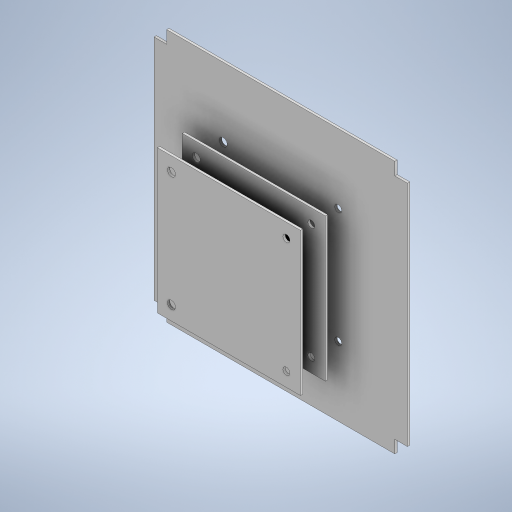
# Autodesk Inventor part: PCB_COM_BAT
Saved by Autodesk Inventor 2024 (Build 280153000, 153)
## iProperties
Created: 2023-06-28
Part Number: PCB_COM_BAT
Material: Genérico
Document SubType Name: Modeling
Designer: Personal
Density: 3.19616 g/cm^3
Appearance: Valor por defecto
Mass: 277 g
Surface Area: 1079.17 cm^2
Volume: 86.6665 cm^3
Author: Personal
Autodesk Inventor part; units mm, degrees
ref_plane "YZ Plane" through (0, 0, 0) normal (1, 0, 0) x (0, 1, 0)
sketch "Boceto1" plane through (0, 0, 0) normal (0, 0, 1) x (1, 0, 0)
  line L0 (-121.9033, -49.2033) -> (40.2033, -49.2033) projected
  line L1 (40.2033, -49.2033) -> (40.2033, -40.2033) projected
  line L2 (40.2033, -40.2033) -> (49.2033, -40.2033) projected
  line L3 (49.2033, -40.2033) -> (49.2033, 121.9033) projected
  line L4 (49.2033, 121.9033) -> (40.2033, 121.9033) projected
  line L5 (40.2033, 121.9033) -> (40.2033, 130.9033) projected
  line L6 (40.2033, 130.9033) -> (-121.9033, 130.9033) projected
  line L7 (-121.9033, 130.9033) -> (-121.9033, 121.9033) projected
  line L8 (-130.9033, 121.9033) -> (-130.9033, -40.2033) projected
  line L9 (-121.9033, 121.9033) -> (-130.9033, 121.9033) projected
  line L10 (-130.9033, -40.2033) -> (-121.9033, -40.2033) projected
  line L11 (-121.9033, -40.2033) -> (-121.9033, -49.2033) projected
  circle A0 centre (0, 0) radius 2.5 projected
  circle A1 centre (-81.7, 0) radius 2.8882 projected
  circle A2 centre (0, 81.7) radius 2.5 projected
  circle A3 centre (-81.7, 81.7) radius 2.8882 projected
  point P0 (0, 0)
extrude "Extrusión2" add sketch "Boceto1" along normal blind 1.65
ref_plane "Plano de trabajo1" through (0, 0, 19.15) normal (0, 0, 1) x (1, 0, 0)
sketch "Boceto2" plane through (0, 0, 19.15) normal (0, 0, 1) x (1, 0, 0)
  line L0 (40.2033, -49.2033) -> (40.2033, -40.2033) construction
  line L1 (40.2033, -40.2033) -> (49.2033, -40.2033) construction
  line L2 (49.2033, -40.2033) -> (49.2033, 121.9033) construction
  line L3 (49.2033, 121.9033) -> (40.2033, 121.9033) construction
  line L4 (40.2033, 121.9033) -> (40.2033, 130.9033) construction
  line L5 (40.2033, 130.9033) -> (-121.9033, 130.9033) construction
  line L6 (-121.9033, 130.9033) -> (-121.9033, 121.9033) construction
  line L7 (-121.9033, 121.9033) -> (-130.9033, 121.9033) construction
  line L8 (-130.9033, 121.9033) -> (-130.9033, -40.2033) construction
  line L9 (-130.9033, -40.2033) -> (-121.9033, -40.2033) construction
  line L10 (-121.9033, -40.2033) -> (-121.9033, -49.2033) construction
  line L11 (-121.9033, -49.2033) -> (40.2033, -49.2033) construction
  circle A0 centre (0, 0) radius 2.5 projected
  circle A1 centre (-81.7, 0) radius 2.8882 projected
  circle A2 centre (0, 81.7) radius 2.5 projected
  circle A3 centre (-81.7, 81.7) radius 2.8882 projected
  line L12 (-91.7016, 91.6984) -> (9.9984, 91.6984)
  line L13 (9.9984, 91.6984) -> (9.9984, -10.0016)
  line L14 (9.9984, -10.0016) -> (-91.7016, -10.0016)
  line L15 (-91.7016, -10.0016) -> (-91.7016, 91.6984)
  line L16 (-91.7016, 91.6984) -> (9.9984, -10.0016) construction
  line L17 (9.9984, 91.6984) -> (-91.7016, -10.0016) construction
  point P0 (0, 0)
  point P1 (-40.8516, 40.8484)
  dimension "d5" = 101.7
  dimension "d6" = 101.7
  dimension "d7" = 39.2049
  dimension "d8" = 39.2017
  dimension "d9" = 39.2049
  constraints: 12 end point, 2 midpoint, 2 parallel, 1 horizontal, 1 perpendicular
  measures "d5" distance of L12.end L13.end
  measures "d6" distance of L13.end L14.end
  measures "d7" distance between parallel lines of L5 L12
  measures "d8" distance between parallel lines of L11 L14
  measures "d9" distance between parallel lines of L2 L13
extrude "Extrusión3" add sketch "Boceto2" along normal blind 1.65
ref_plane "Plano de trabajo2" through (0, 0, 36.8) normal (0, 0, 1) x (1, 0, 0)
sketch "Boceto3" plane through (0, 0, 36.8) normal (0, 0, 1) x (1, 0, 0)
  line L0 (-91.7016, -10.0016) -> (9.9984, -10.0016) projected
  line L1 (9.9984, -10.0016) -> (9.9984, 91.6984) projected
  line L2 (9.9984, 91.6984) -> (-91.7016, 91.6984) projected
  line L3 (-91.7016, 91.6984) -> (-91.7016, -10.0016) projected
  circle A0 centre (-81.7, 81.7) radius 2.8882 projected
  circle A1 centre (0, 81.7) radius 2.5 projected
  circle A2 centre (-81.7, 0) radius 2.8882 projected
  circle A3 centre (0, 0) radius 2.5 projected
  point P0 (0, 0)
extrude "Extrusión4" add sketch "Boceto3" along normal blind 1.65
